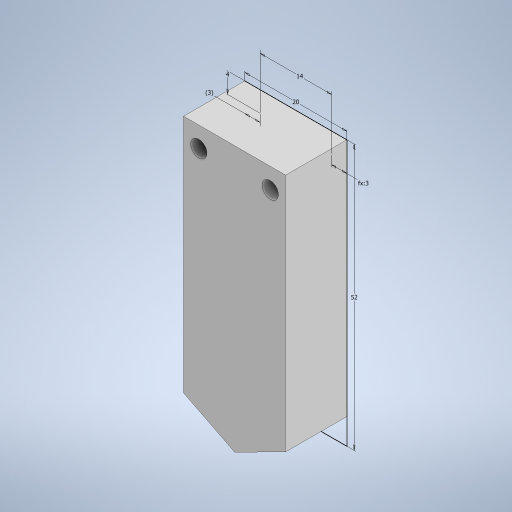
# Autodesk Inventor part: hotend
Saved by Autodesk Inventor 2023.1 (Build 271208000, 208)
## iProperties
Created: 2022-11-02
Part Number: hotend
Material: Generic
Document SubType Name: Modeling
Designer: nicol
Density: 1 g/cm^3
Appearance: Default
Author: nicol
Autodesk Inventor part; units mm, degrees
ref_plane "YZ Plane" through (0, 0, 0) normal (1, 0, 0) x (0, 1, 0)
ref_plane "XZ Plane" through (0, 0, 0) normal (0, 1, 0) x (-1, 0, 0)
ref_plane "XY Plane" through (0, 0, 0) normal (0, 0, 1) x (1, 0, 0)
sketch "Sketch1" plane through (0, 0, 0) normal (0, 0, 1) x (1, 0, 0)
  line L0 (0, 0) -> (20, 0)
  line L1 (20, 0) -> (20, 52)
  line L2 (20, 52) -> (0, 52)
  line L3 (0, 52) -> (0, 0)
  line L4 (10, 0) -> (20, 5.0421)
  line L5 (10, 0) -> (0, 5.0421)
  point P0 (3, 48)
  point P1 (17, 48)
  dimension "d0" = 20
  dimension "d1" = 52
  dimension "d2" = 14
  dimension "d3" = 3
  dimension "d4" = 3
  dimension "d5" = 4
  constraints: 12 end point, 2 parallel, 2 point on line, 1 equal length, 1 horizontal, 1 horizontal alignment, 1 midpoint, 1 perpendicular
  measures "d0" distance of L2.end L1.end
  measures "d1" distance of L1.end L0.end
  measures "d2" distance of point (3, 48) point (17, 48)
  measures "d3" distance from line of L1 point (17, 48)
  measures "d4" distance from line of point (3, 48) L3
  measures "d5" distance from line of L2 point (3, 48)
extrude "Extrusion1" add sketch "Sketch1" along normal blind 12 contours L5 L3 L2 L1 L4
hole "Hole1" at (3, 48, 0) at (17, 48, 0) direction (0, 0, 1) diameter 3.2 end through all
equation "\"d3\" = d4"
body "Solid1"
